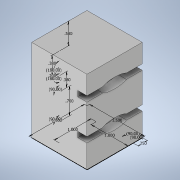
# Autodesk Inventor part: Valve Holder
Saved by Autodesk Inventor 2020 (Build 240168000, 168)
## iProperties
Created: 2022-01-25
Part Number: Valve Holder
Material: Generic
Document SubType Name: Modeling
Designer: Beaucage
Density: 1 g/cm^3
Appearance: Default
Author: Beaucage
Autodesk Inventor part; units mm, degrees
ref_plane "YZ Plane" through (0, 0, 0) normal (1, 0, 0) x (0, 1, 0)
ref_plane "XZ Plane" through (0, 0, 0) normal (0, 1, 0) x (-1, 0, 0)
ref_plane "XY Plane" through (0, 0, 0) normal (0, 0, 1) x (1, 0, 0)
sketch "Sketch1" plane through (0, 0, 0) normal (0, 1, 0) x (-1, 0, 0)
  line L0 (0, 0) -> (38.1, 0)
  line L1 (38.1, 0) -> (38.1, -38.1)
  line L2 (38.1, -38.1) -> (0, -38.1)
  line L3 (0, -38.1) -> (0, 0)
  line L4 (0, -38.1) -> (0, -31.75)
  line L5 (0, -38.1) -> (6.35, -38.1) construction
  line L6 (0, -31.75) -> (25.4, -31.75)
  line L7 (25.4, -31.75) -> (25.4, -6.35)
  dimension "d0" = 38.1
  dimension "d1" = 38.1
  dimension "d2" = 6.35
  dimension "d3" = 90
  dimension "d4" = 25.4
  dimension "d5" = 90
  dimension "d6" = 25.4
  constraints: 16 end point, 4 perpendicular, 2 horizontal, 2 parallel, 1 collinear
  measures "d0" distance of L1.end L2.end
  measures "d1" distance of L0.end L1.end
  measures "d2" distance of L2.end L4.end
  measures "d3" angle of L5 L4
  measures "d4" distance of L4.end L6.end
  measures "d5" angle of L4 L6
  measures "d6" distance of L6.end L7.end
extrude "Extrusion1" add sketch "Sketch1" along normal blind 56.896
hole "Hole1" at (-25.4, 0, -31.75) at (-25.4, 0, -6.35) direction (0, 1, 0) diameter 7.9375 depth 12.7
sketch "Sketch2" plane through (-38.1, 0, -38.1) normal (-1, 0, 0) x (0, 0, 1)
  line L0 (38.1, 0) -> (0, 0) projected
  line L1 (19.05, 0) -> (19.05, 17.78)
  line L2 (19.05, 0) -> (36.83, 0) construction
  line L3 (19.05, 17.78) -> (19.05, 27.432)
  line L4 (19.05, 17.78) -> (28.702, 17.78) construction
  line L5 (19.05, 27.432) -> (19.05, 32.512)
  line L6 (19.05, 32.512) -> (19.05, 42.164)
  circle A0 centre (19.05, 17.78) radius 9.652
  circle A1 centre (19.05, 42.164) radius 9.652
  ellipse E0 centre (19.05, 42.164) end of major axis (28.702, 42.164) minor radius 3.5267
  ellipse E1 centre (19.05, 17.78) end of major axis (28.702, 17.78) minor radius 3.6751
  line L7 (19.05, 42.164) -> (19.05, 56.896)
  dimension "d16" = 17.78
  dimension "d17" = 90
  dimension "d18" = 9.652
  dimension "d19" = 90
  dimension "d20" = 5.08
  dimension "d21" = 180
  dimension "d22" = 9.652
  dimension "d23" = 180
  dimension "d32" = 14.732
  constraints: 14 end point, 4 coincident, 3 horizontal, 3 vertical, 2 collinear, 2 perpendicular, 2 vertical alignment, 1 centre point, 1 horizontal alignment, 1 line through centre, 1 midpoint, 6 other
  measures "d16" distance of L1.start L1.end
  measures "d17" angle of L2 L1
  measures "d18" distance of L1.end L3.end
  measures "d19" angle of L4 L3
  measures "d20" distance of L3.end L5.end
  measures "d21" angle of L5 L3
  measures "d22" distance of L5.end L6.end
  measures "d23" angle of L6 L5
  measures "d32" distance of L7.start L7.end
extrude "Extrusion2" cut sketch "Sketch2" against normal blind 31.75
extrude "Extrusion3" cut sketch "Sketch2" against normal blind 38.1 contours E1 L3 L1 | L1 L3 E1 | E0 L7 L6 | L6 L7 E0
sketch "Sketch3" plane through (0, 0, 0) normal (1, 0, 0) x (0, 0, -1)
  line L0 (38.1, 0) -> (38.1, 56.896) projected
  line L1 (0, 44.069) -> (38.1, 44.069)
  line L2 (38.1, 44.069) -> (38.1, 40.259)
  line L3 (38.1, 40.259) -> (0, 40.259)
  line L4 (0, 40.259) -> (0, 44.069)
  line L5 (0, 44.069) -> (38.1, 40.259) construction
  line L6 (38.1, 44.069) -> (0, 40.259) construction
  line L7 (0, 19.685) -> (38.1, 19.685)
  line L8 (38.1, 19.685) -> (38.1, 15.875)
  line L9 (38.1, 15.875) -> (0, 15.875)
  line L10 (0, 15.875) -> (0, 19.685)
  line L11 (0, 19.685) -> (38.1, 15.875) construction
  line L12 (38.1, 19.685) -> (0, 15.875) construction
  point P0 (0, 0)
  point P1 (19.05, 17.78)
  point P2 (19.05, 42.164)
  dimension "d28" = 3.81
  dimension "d29" = 3.81
  constraints: 24 end point, 4 midpoint, 4 parallel, 2 horizontal, 2 perpendicular, 2 point on line
  measures "d28" distance of L1.end L2.end
  measures "d29" distance of L7.end L8.end
extrude "Extrusion4" cut sketch "Sketch3" against normal blind 6.35
body "Solid1"
